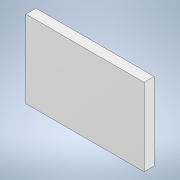
# Autodesk Inventor part: tray
Saved by Autodesk Inventor 2021.1 (Build 251245010, 245A)
## iProperties
Created: 2021-07-04
Part Number: tray
Material: PVC, Unplasticized
Document SubType Name: Modeling
Designer: hp
Density: 1.29 g/cm^3
Appearance: Smooth - White
Author: hp
Autodesk Inventor part; units mm, degrees
ref_plane "YZ Plane" through (0, 0, 0) normal (1, 0, 0) x (0, 1, 0)
ref_plane "XZ Plane" through (0, 0, 0) normal (0, 1, 0) x (-1, 0, 0)
ref_plane "XY Plane" through (0, 0, 0) normal (0, 0, 1) x (1, 0, 0)
sketch "Sketch1" plane through (0, 0, 0) normal (0, 0, 1) x (1, 0, 0)
  line L0 (145, 95) -> (-145, 95)
  line L1 (-145, 95) -> (-145, -95)
  line L2 (-145, -95) -> (145, -95)
  line L3 (145, -95) -> (145, 95)
  line L4 (145, 95) -> (-145, -95) construction
  line L5 (-145, 95) -> (145, -95) construction
  point P0 (0, 0)
  dimension "d0" = 290
  dimension "d1" = 190
  constraints: 12 end point, 2 midpoint, 2 parallel, 1 horizontal, 1 perpendicular
  measures "d0" distance of L0.start L0.end
  measures "d1" distance of L2.end L0.start
extrude "Extrusion1" add sketch "Sketch1" along normal blind 25
shell "Shell1" thickness 1 removed faces 1 at (-48.3333, -31.6667, 0)
body "Solid1"
